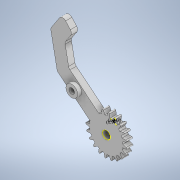
# Autodesk Inventor part: Servo pinza 2
Saved by Autodesk Inventor 2021 (Build 250183000, 183)
## iProperties
Created: 2021-03-24
Part Number: Servo pinza 2
Material: Generic
Document SubType Name: Modeling
Designer: LCG
Density: 1 g/cm^3
Appearance: Default
Author: LCG
Autodesk Inventor part; units mm, degrees
ref_plane "YZ Plane" through (0, 0, 0) normal (1, 0, 0) x (0, 1, 0)
ref_plane "XZ Plane" through (0, 0, 0) normal (0, 1, 0) x (-1, 0, 0)
ref_plane "XY Plane" through (0, 0, 0) normal (0, 0, 1) x (1, 0, 0)
sketch "Sketch1" plane through (0, 0, 0) normal (0, 0, 1) x (1, 0, 0)
  circle A0 centre (0, 0) radius 2.5
  line L0 (0, 0) -> (-15.5714, 12.5511)
  line L1 (0, 0) -> (20, 0) construction
  line L2 (-15.5714, 12.5511) -> (-18.3421, 9.1137)
  line L3 (0, 0) -> (-10.3273, 2.6535)
  line L4 (0, 0) -> (26.0413, 0) construction
  line L5 (-18.3421, 9.1137) -> (-10.3273, 2.6535)
  line L6 (-23.1447, 24.3261) -> (-21.5758, 26.2725)
  circle A1 centre (-21.5758, 26.2725) radius 2.5
  line L7 (-23.6708, 23.9703) -> (-17.7415, 23.9703) construction
  line L8 (-24.0288, 25.7899) -> (-26.2178, 36.9166)
  line L9 (-24.0288, 25.7899) -> (-12.6888, 25.7899) construction
  line L10 (-26.2178, 36.9166) -> (-23.7649, 37.3992)
  circle A2 centre (-23.7649, 37.3992) radius 2.5
  line L11 (-26.2069, 38.2378) -> (-20.9991, 38.2378) construction
  line L12 (-25.8513, 38.7765) -> (-22.6835, 43.5752)
  line L13 (-25.8513, 38.7765) -> (-20.1013, 38.7765) construction
  line L14 (-22.6835, 43.5752) -> (-24.7699, 44.9525)
  circle A3 centre (-24.7699, 44.9525) radius 2.5
  line L15 (0, 0) -> (60, 0) construction
  line L16 (-25.9313, 49.9817) -> (-22.9112, 46.6245)
  line L17 (-24.7699, 40.4146) -> (-32.5897, 45.5767)
  line L18 (-32.5897, 45.5767) -> (-29.8763, 49.6871)
  line L19 (-32.5897, 45.5767) -> (-34.946, 42.0073)
  line L20 (-25.1233, 31.3533) -> (-33.2672, 29.7511)
  line L21 (-33.2672, 29.7511) -> (-35.3126, 40.1474)
  line L22 (-33.2672, 29.7511) -> (-31.4304, 20.4146)
  line L23 (-18.3421, 9.1137) -> (-30.5463, 18.9507)
  line L24 (-16.7222, 19.1493) -> (-22.2635, 12.2745)
  arc A4 (-10.3273, 2.6535) -> (-4.786, 9.5283) centre (0, 0) ccw
  arc A5 (-25.9313, 49.9817) -> (-29.8763, 49.6871) centre (-27.7899, 48.3098) ccw
  arc A6 (-34.946, 42.0073) -> (-35.3126, 40.1474) centre (-32.8596, 40.63) ccw
  arc A7 (-31.4304, 20.4146) -> (-30.5463, 18.9507) centre (-28.9774, 20.8971) ccw
  line L25 (-16.7222, 19.1493) -> (-23.1447, 24.3261)
  line L26 (-16.7222, 19.1493) -> (-4.786, 9.5283)
  circle A8 centre (-19.4928, 15.7119) radius 1.75
  line L27 (0, 0) -> (-10.6628, 0)
  line L28 (-4.786, 9.5283) -> (0, 0)
  arc A9 (-12.7774, 0.4964) -> (-12.7774, -0.4964) centre (-12.6628, 0) ccw
  line L29 (-10.6628, 0) -> (-10.1628, 0)
  line L30 (-10.6162, 0.9953) -> (-12.7774, 0.4964)
  line L31 (-10.6162, -0.9953) -> (-12.7774, -0.4964)
  line L32 (-10.4242, -2.2431) -> (-12.3353, -3.3688)
  line L33 (-9.8256, -4.1416) -> (-12.0367, -4.3157)
  arc A10 (-12.3353, -3.3688) -> (-12.0367, -4.3157) centre (-12.0767, -3.8078) ccw
  line L34 (-9.2672, -5.2739) -> (-10.7513, -6.9222)
  line L35 (-8.1254, -6.9045) -> (-10.1819, -7.7354)
  arc A11 (-10.7513, -6.9222) -> (-10.1819, -7.7354) centre (-10.3727, -7.2631) ccw
  line L36 (-7.2524, -7.8165) -> (-8.1722, -9.8348)
  line L37 (-5.6731, -9.0283) -> (-7.3845, -10.4392)
  arc A12 (-8.1722, -9.8348) -> (-7.3845, -10.4392) centre (-7.7086, -10.046) ccw
  line L38 (-4.5663, -9.6356) -> (-4.8366, -11.837)
  line L39 (-2.6957, -10.3164) -> (-3.9036, -12.1766)
  arc A13 (-4.8366, -11.837) -> (-3.9036, -12.1766) centre (-4.3309, -11.8991) ccw
  line L40 (-1.4574, -10.5627) -> (-1.0533, -12.7435)
  line L41 (0.5313, -10.6495) -> (-0.0614, -12.7869)
  arc A14 (-1.0533, -12.7435) -> (-0.0614, -12.7869) centre (-0.5523, -12.6507) ccw
  line L42 (1.7863, -10.5121) -> (2.8275, -12.4705)
  line L43 (3.7091, -9.9969) -> (3.7865, -12.2135)
  arc A15 (2.8275, -12.4705) -> (3.7865, -12.2135) centre (3.2774, -12.2313) ccw
  line L44 (4.8646, -9.4884) -> (6.4466, -11.043)
  line L45 (6.5435, -8.4188) -> (7.2839, -10.5096)
  arc A16 (6.4466, -11.043) -> (7.2839, -10.5096) centre (6.8037, -10.6797) ccw
  line L46 (7.4927, -7.5864) -> (9.4689, -8.5934)
  line L47 (8.7723, -6.0615) -> (10.1071, -7.8329)
  arc A17 (9.4689, -8.5934) -> (10.1071, -7.8329) centre (9.7002, -8.1395) ccw
  line L48 (9.4272, -4.9822) -> (11.6148, -5.3483)
  line L49 (10.189, -3.1431) -> (11.9947, -4.4311)
  arc A18 (11.6148, -5.3483) -> (11.9947, -4.4311) centre (11.6989, -4.8458) ccw
  line L50 (10.4891, -1.9168) -> (12.6855, -1.6081)
  line L51 (10.6626, 0.0663) -> (12.772, -0.6191)
  arc A19 (12.6855, -1.6081) -> (12.772, -0.6191) centre (12.6146, -1.1036) ccw
  line L52 (10.58, 1.326) -> (12.5819, 2.2809)
  line L53 (10.1491, 3.2695) -> (12.367, 3.2502)
  arc A20 (12.5819, 2.2809) -> (12.367, 3.2502) centre (12.3626, 2.7407) ccw
  line L54 (9.6916, 4.4461) -> (11.3137, 5.9588)
  line L55 (8.6962, 6.1701) -> (10.8173, 6.8186)
  arc A21 (11.3137, 5.9588) -> (10.8173, 6.8186) centre (10.9663, 6.3314) ccw
  line L56 (7.906, 7.1547) -> (8.9982, 9.0851)
  line L57 (6.4384, 8.4995) -> (8.2663, 9.7558)
  arc A22 (8.9982, 9.0851) -> (8.2663, 9.7558) centre (8.5548, 9.336) ccw
  line L58 (5.3887, 9.2009) -> (5.8498, 11.3704)
  line L59 (3.5845, 10.0422) -> (4.9501, 11.79)
  arc A23 (5.8498, 11.3704) -> (4.9501, 11.79) centre (5.3515, 11.4764) ccw
  line L60 (2.3725, 10.3955) -> (2.1599, 12.6033)
  line L61 (0.3989, 10.6553) -> (1.1756, 12.7328)
  arc A24 (2.1599, 12.6033) -> (1.1756, 12.7328) centre (1.6528, 12.5544) ccw
  line L62 (-0.8633, 10.6278) -> (-1.7299, 12.6694)
  line L63 (-2.8237, 10.2821) -> (-2.7076, 12.497)
  arc A25 (-1.7299, 12.6694) -> (-2.7076, 12.497) centre (-2.1989, 12.4704) ccw
  point P0 (-10.1693, -3.2064)
  point P1 (-8.7344, -6.1159)
  point P2 (-6.4911, -8.4593)
  point P3 (-3.6469, -10.0197)
  point P4 (-0.4651, -10.6526)
  point P5 (2.7597, -10.2994)
  point P6 (5.7291, -8.9929)
  point P7 (8.1681, -6.8539)
  point P8 (9.8511, -4.0805)
  point P9 (10.6222, -0.9293)
  point P10 (10.41, 2.3078)
  point P11 (9.2342, 5.3314)
  point P12 (7.2037, 7.8614)
  point P13 (4.5063, 9.6637)
  point P14 (1.3918, 10.5715)
  point P15 (-1.8516, 10.5008)
  dimension "d0" = 5
  dimension "d1" = 20
  dimension "d2" = 141.13
  dimension "d3" = 4.415
  dimension "d4" = 165.59
  dimension "d6" = 10.2942
  dimension "d8" = 2.5
  dimension "d11" = 11.34
  dimension "d13" = 101.13
  dimension "d14" = 2.5
  dimension "d16" = 5.75
  dimension "d17" = 56.57
  dimension "d18" = 2.5
  dimension "d22" = 9.37
  dimension "d23" = 8.3
  dimension "d25" = 8.83
  dimension "d26" = 2.5
  dimension "d27" = 3.5
  dimension "d34" = 63.33
  dimension "d41" = 0.5
  dimension "d46" = 280
  constraints: 128 end point, 44 point on circle, 24 centre point, 12 perpendicular, 10 tangent, 7 horizontal, 5 coincident, 4 point on line, 3 equal length, 2 equal radius, 2 midpoint, 157 other
  measures "d0" diameter of A0
  measures "d1" distance of L0.start L0.end
  measures "d2" angle of L1 L0
  measures "d3" distance of L0.end L2.end
  measures "d4" angle of L4 L3
  measures "d6" distance of L3.end L2.end
  measures "d8" distance of L6.start L6.end
  measures "d11" distance of L8.start L8.end
  measures "d13" angle of L9 L8
  measures "d14" distance of L8.end L10.end
  measures "d16" distance of L12.start L12.end
  measures "d17" angle of L13 L12
  measures "d18" distance of L12.end L14.end
  measures "d22" distance of L17.start L17.end
  measures "d23" distance of L20.start L20.end
  measures "d25" distance of L24.start L24.end
  measures "d26" radius of A5
  measures "d27" diameter of A8
  measures "d34" angle of L28 L27
  measures "d41" distance of L27.end L29.end
extrude "Extrusion1" add sketch "Sketch1" along normal blind 4 contours A0 L28 A4 L27 | A0 L0 L2 L23 L24 A8 L26 L28 | L27 A4 L3 A0 | A0 L3 L5 L2 L0 | L63 A25 L62 A4 | L24 A8 L23 A7 L22 L20 L8 A1 L25 | A4 L31 A9 L30 | L61 A24 L60 A4 | A4 L33 A10 L32 | L20 L21 A6 L19 L17 L12 A2 L8 | L59 A23 L58 A4 | A4 L35 A11 L34 | L57 A22 L56 A4 | L17 L18 A5 L16 A3 L12 | A4 L37 A12 L36 | A3 | L55 A21 L54 A4 | A4 L39 A13 L38 | L53 A20 L52 A4 | A4 L41 A14 L40 | L51 A19 L50 A4 | A4 L43 A15 L42 | L49 A18 L48 A4 | A4 L45 A16 L44 | L47 A17 L46 A4
sketch "Sketch2" plane through (0, 0, 4) normal (0, 0, 1) x (1, 0, 0)
  circle A0 centre (-19.4928, 15.7119) radius 1.75 projected
  circle A1 centre (-19.4928, 15.7119) radius 1.75
  circle A2 centre (-19.4928, 15.7119) radius 3.75
  point P0 (0, 0)
  dimension "d50" = 7.5
  constraints: 2 centre point, 2 coincident
  measures "d50" diameter of A2
extrude "Extrusion2" add sketch "Sketch2" along normal blind 2.5
sketch "Sketch3" plane through (0, 0, 4) normal (0, 0, 1) x (1, 0, 0)
  circle A0 centre (0, 0) radius 2.5 projected
  arc A1 (3.5845, 10.0422) -> (2.3725, 10.3955) centre (0, 0) ccw projected
  arc A2 (6.4384, 8.4995) -> (5.3887, 9.2009) centre (0, 0) ccw projected
  line L0 (3.5845, 10.0422) -> (5.3887, 9.2009)
  arc A3 (5.8498, 11.3704) -> (4.9501, 11.79) centre (5.3515, 11.4764) ccw projected
  line L1 (4.4866, 9.6215) -> (5.3515, 11.4764)
  dimension "d53" = 1.9906
  dimension "d54" = 2.0466
  constraints: 4 end point, 1 midpoint
  measures "d53" distance of L0.start L0.end
  measures "d54" distance of L1.start L1.end
body "Solid1"
